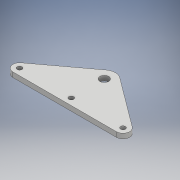
# Autodesk Inventor part: Corpo_Suporte_3_Cabos_Modelo1
Saved by Autodesk Inventor 2018 (Build 220112000, 112)
## iProperties
Created: 2021-08-02
Part Number: Corpo_Suporte_3_Cabos_Modelo1
Material: Generic
Document SubType Name: Modeling
Designer: L08619
Density: 1 g/cm^3
Appearance: Default
Author: L08619
Autodesk Inventor part; units mm, degrees
ref_plane "YZ Plane" through (0, 0, 0) normal (1, 0, 0) x (0, 1, 0)
ref_plane "XZ Plane" through (0, 0, 0) normal (0, 1, 0) x (-1, 0, 0)
ref_plane "XY Plane" through (0, 0, 0) normal (0, 0, 1) x (1, 0, 0)
sketch "Sketch1" plane through (0, 0, 0) normal (0, 0, 1) x (1, 0, 0)
  circle A0 centre (0, 0) radius 20
  circle A1 centre (-235, -150) radius 11
  circle A2 centre (0, -150) radius 11
  arc A3 (-252.9136, -125.9354) -> (-235, -180) centre (-235, -150) ccw
  line L0 (0, 87.1559) -> (0, -290.9336) construction
  circle A4 centre (235, -150) radius 11
  arc A5 (235, -180) -> (252.9136, -125.9354) centre (235, -150) ccw
  line L1 (-235, -180) -> (235, -180)
  arc A6 (29.8559, 40.1076) -> (-29.8559, 40.1076) centre (0, 0) ccw
  line L2 (-252.9136, -125.9354) -> (-29.8559, 40.1076)
  line L3 (252.9136, -125.9354) -> (29.8559, 40.1076)
  point P0 (0, -180)
  point P1 (0, 46.2314)
  dimension "d0" = 40
  dimension "d1" = 22
  dimension "d3" = 22
  dimension "d4" = 150
  dimension "d8" = 235
  dimension "d16" = 470
  dimension "d17" = 30
  dimension "d18" = 100
  constraints: 8 end point, 7 centre point, 6 point on circle, 5 tangent, 4 coincident, 3 symmetric about line, 2 point on line, 1 horizontal, 1 horizontal alignment, 1 vertical, 1 vertical alignment, 2 other
  measures "d0" diameter of A0
  measures "d1" diameter of A2
  measures "d3" diameter of A1
  measures "d4" distance of point (0, 0) A2.centre
  measures "d8" distance of A2.centre A1.centre
  measures "d16" distance of A4.centre A1.centre
  measures "d17" radius of A5
  measures "d18" diameter of A6
extrude "Extrusion1" add sketch "Sketch1" along normal mid plane 22.22
equation "\"d1\" = d3"
body "Solid1"
